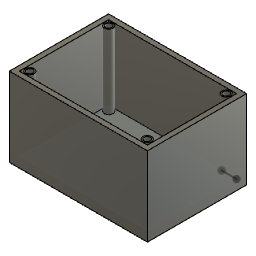
SmartEFM_BS v11 (Autodesk Fusion 360 design; units mm, degrees)
Autodesk Fusion 360 part; units mm, degrees
sketch "Sketch1" plane through (0, 0, 0) normal (0, 1, 0) x (1, 0, 0)
  line L0 (0, 0) -> (110, 0)
  line L1 (110, 0) -> (110, -79)
  line L2 (110, -79) -> (0, -79)
  line L3 (0, -79) -> (0, 0)
  dimension "d1" = 110
  dimension "d2" = 79
  constraint horizontal L0
  constraint vertical L1
  constraint horizontal L2
  constraint vertical L3
  constraint coincident L0.start L3.end
  measures "d1" distance of L0.start L0.end
  measures "d2" distance of L0.start L2.end
extrude "Extrude1" add sketch "Sketch1" along normal blind 63
shell "Shell1" thickness 4 removed faces 1 at (36.6667, 63, 52.6667)
sketch "Sketch2" plane through (0, 4, 0) normal (0, 1, 0) x (-1, 0, 0)
  line L0 (-4, 75) -> (-106, 75)
  line L1 (-106, 75) -> (-106, 4)
  line L2 (-106, 4) -> (-4, 4)
  line L3 (-4, 4) -> (-4, 75)
  line L4 (-106, 4) -> (-94.15, 4)
  dimension "d6" = 11.85
  constraint coincident L1.end L2.start
  constraint perpendicular L1 L4
  measures "d6" distance of L1.end L4.end
sketch "Sketch3" plane through (0, 0, 4) normal (0, 0, 1) x (1, 0, 0)
  line L0 (4, 4) -> (106, 4)
  line L1 (106, 4) -> (106, 63)
  line L2 (106, 63) -> (4, 63)
  line L3 (4, 63) -> (4, 4)
  line L4 (94.2648, 4) -> (94.2648, 15)
  line L5 (94.2648, 15) -> (85, 15)
  line L6 (85, 15) -> (85, 4)
  constraint coincident L0 L4.start
  constraint perpendicular L0 L4
  constraint perpendicular L4 L5
  constraint coincident L0 L6.end
  constraint perpendicular L0 L6
extrude "Extrude2" cut sketch "Sketch3" against normal blind 10 contours L0 L4 L5 L6
sketch "Sketch4" plane through (55, 4, 39.5) normal (0, 1, 0) x (-1, 0, 0)
  line L0 (50, 0) -> (-40, 0)
  line L1 (0, 35) -> (0, -30)
  circle A0 centre (46.8265, 31.4383) radius 3.5
  circle A1 centre (-46.8265, 31.4383) radius 3.5
  circle A2 centre (46.8265, -31.4383) radius 3.5
  circle A3 centre (-46.8265, -31.4383) radius 3.5
  dimension "d9" = 7
  constraint horizontal L0
  constraint perpendicular L0 L1
  constraint symmetric L1 A0 A1
  constraint symmetric L0 A0 A2
  constraint symmetric L1 A2 A3
  measures "d9" diameter of A0
extrude "Extrude3" add sketch "Sketch4" along normal blind 59
hole "Hole1" at (101.8265, 63, 70.9383) direction (0, -1, 0) diameter 5 depth 40 tip angle 118
hole "Hole2" at (101.8584, 63, 8.0262) direction (0, -1, 0) diameter 5 depth 40 tip angle 118
hole "Hole3" at (8.1695, 63, 8.0613) direction (0, -1, 0) diameter 5 depth 40 tip angle 118
hole "Hole4" at (8.1735, 63, 70.9383) direction (0, -1, 0) diameter 5 depth 40 tip angle 118
